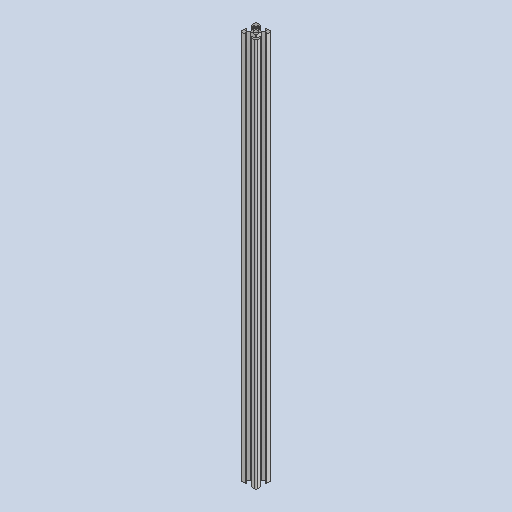
# Autodesk Inventor part: HCMUTE-CDT23-OP_NDH-2020X500
Saved by Autodesk Inventor 2023 (Build 270158000, 158)
## iProperties
Created: 2023-11-14
Part Number: HCMUTE-CDT23-OP_NDH-2020X500
Material: Generic
Document SubType Name: Modeling
Designer: havie
Density: 1 g/cm^3
Appearance: Default
Author: havie
Autodesk Inventor part; units mm, degrees
ref_plane "YZ Plane" through (0, 0, 0) normal (1, 0, 0) x (0, 1, 0)
ref_plane "XZ Plane" through (0, 0, 0) normal (0, 1, 0) x (-1, 0, 0)
ref_plane "XY Plane" through (0, 0, 0) normal (0, 0, 1) x (1, 0, 0)
sketch "Sketch1" plane through (0, 0, 0) normal (0, 0, 1) x (1, 0, 0)
  line L0 (-8.5, 10) -> (-4.1, 10)
  line L1 (10, 10) -> (10, -10)
  line L2 (10, -10) -> (-10, -10)
  line L3 (-10, 4.1) -> (-10, 8.5)
  line L4 (-10, 10) -> (10, -10) construction
  line L5 (10, 10) -> (-10, -10) construction
  line L6 (2.9101, 3.9) -> (-2.9101, 3.9)
  line L7 (-3.9, 2.9101) -> (-3.9, -2.9101)
  line L8 (3.9, -2.9101) -> (3.9, 2.9101)
  line L9 (-3.1, 9) -> (-3.1, 8.7)
  line L10 (-3.6, 8.2) -> (-5, 8.2)
  line L11 (-5.5, 7.7) -> (-5.5, 6.4899)
  line L12 (-8.2, 5) -> (-8.2, 3.6)
  line L13 (-8.7, 3.1) -> (-9, 3.1)
  line L14 (-7.7, 5.5) -> (-6.4899, 5.5)
  arc A0 (-8.5, 10) -> (-10, 8.5) centre (-8.5, 8.5) ccw
  line L15 (-3.6, 9.5) -> (-3.6, 9.5)
  line L16 (-3.6, 9.5) -> (-3.6, 9.5)
  line L17 (-9.5, 3.6) -> (-9.5, 3.6)
  line L18 (-9.5, 3.6) -> (-9.5, 3.6)
  arc A1 (-5, 8.2) -> (-5.5, 7.7) centre (-5, 7.7) ccw
  arc A2 (-7.7, 5.5) -> (-8.2, 5) centre (-7.7, 5) ccw
  arc A3 (-8.7, 3.1) -> (-8.2, 3.6) centre (-8.7, 3.6) ccw
  arc A4 (-3.6, 8.2) -> (-3.1, 8.7) centre (-3.6, 8.7) ccw
  arc A5 (-3.1, 9) -> (-3.6, 9.5) centre (-3.6, 9) ccw
  arc A6 (-3.6, 9.5) -> (-4.1, 10) centre (-4.1, 9.5) ccw
  arc A7 (-9.5, 3.6) -> (-9, 3.1) centre (-9, 3.6) ccw
  arc A8 (-10, 4.1) -> (-9.5, 3.6) centre (-9.5, 4.1) ccw
  line L19 (-6.4899, 5.5) -> (-3.9, 2.9101)
  line L20 (-5.5, 6.4899) -> (-2.9101, 3.9)
  line L21 (-14.4349, 0) -> (14.4349, 0) construction
  line L22 (0, -14.4349) -> (0, 14.4349) construction
  line L23 (8.5, 10) -> (4.1, 10)
  line L24 (10, 4.1) -> (10, 8.5)
  line L25 (3.1, 9) -> (3.1, 8.7)
  line L26 (3.6, 8.2) -> (5, 8.2)
  line L27 (5.5, 7.7) -> (5.5, 6.4899)
  line L28 (8.2, 5) -> (8.2, 3.6)
  line L29 (8.7, 3.1) -> (9, 3.1)
  line L30 (7.7, 5.5) -> (6.4899, 5.5)
  arc A9 (10, 8.5) -> (8.5, 10) centre (8.5, 8.5) ccw
  line L31 (3.6, 9.5) -> (3.6, 9.5)
  line L32 (3.6, 9.5) -> (3.6, 9.5)
  line L33 (9.5, 3.6) -> (9.5, 3.6)
  line L34 (9.5, 3.6) -> (9.5, 3.6)
  arc A10 (5.5, 7.7) -> (5, 8.2) centre (5, 7.7) ccw
  arc A11 (8.2, 5) -> (7.7, 5.5) centre (7.7, 5) ccw
  arc A12 (8.2, 3.6) -> (8.7, 3.1) centre (8.7, 3.6) ccw
  arc A13 (3.1, 8.7) -> (3.6, 8.2) centre (3.6, 8.7) ccw
  arc A14 (3.6, 9.5) -> (3.1, 9) centre (3.6, 9) ccw
  arc A15 (4.1, 10) -> (3.6, 9.5) centre (4.1, 9.5) ccw
  arc A16 (9, 3.1) -> (9.5, 3.6) centre (9, 3.6) ccw
  arc A17 (9.5, 3.6) -> (10, 4.1) centre (9.5, 4.1) ccw
  line L35 (6.4899, 5.5) -> (3.9, 2.9101)
  line L36 (5.5, 6.4899) -> (2.9101, 3.9)
  line L37 (-8.5, -10) -> (-4.1, -10)
  line L38 (-10, -4.1) -> (-10, -8.5)
  line L39 (-3.1, -9) -> (-3.1, -8.7)
  line L40 (-3.6, -8.2) -> (-5, -8.2)
  line L41 (-5.5, -7.7) -> (-5.5, -6.4899)
  line L42 (-8.2, -5) -> (-8.2, -3.6)
  line L43 (-8.7, -3.1) -> (-9, -3.1)
  line L44 (-7.7, -5.5) -> (-6.4899, -5.5)
  arc A18 (-10, -8.5) -> (-8.5, -10) centre (-8.5, -8.5) ccw
  arc A19 (-5.5, -7.7) -> (-5, -8.2) centre (-5, -7.7) ccw
  arc A20 (-8.2, -5) -> (-7.7, -5.5) centre (-7.7, -5) ccw
  arc A21 (-8.2, -3.6) -> (-8.7, -3.1) centre (-8.7, -3.6) ccw
  arc A22 (-3.1, -8.7) -> (-3.6, -8.2) centre (-3.6, -8.7) ccw
  arc A23 (-3.6, -9.5) -> (-3.1, -9) centre (-3.6, -9) ccw
  arc A24 (-4.1, -10) -> (-3.6, -9.5) centre (-4.1, -9.5) ccw
  arc A25 (-9, -3.1) -> (-9.5, -3.6) centre (-9, -3.6) ccw
  arc A26 (-9.5, -3.6) -> (-10, -4.1) centre (-9.5, -4.1) ccw
  line L45 (-6.4899, -5.5) -> (-3.9, -2.9101)
  line L46 (-5.5, -6.4899) -> (-2.9101, -3.9)
  arc A27 (10, -4.1) -> (9.5, -3.6) centre (9.5, -4.1) ccw
  line L47 (6.4899, -5.5) -> (3.9, -2.9101)
  arc A28 (7.7, -5.5) -> (8.2, -5) centre (7.7, -5) ccw
  line L48 (5.5, -7.7) -> (5.5, -6.4899)
  line L49 (10, -4.1) -> (10, -8.5)
  line L50 (3.1, -9) -> (3.1, -8.7)
  line L51 (8.5, -10) -> (4.1, -10)
  line L52 (3.6, -8.2) -> (5, -8.2)
  arc A29 (5, -8.2) -> (5.5, -7.7) centre (5, -7.7) ccw
  line L53 (7.7, -5.5) -> (6.4899, -5.5)
  arc A30 (8.7, -3.1) -> (8.2, -3.6) centre (8.7, -3.6) ccw
  arc A31 (8.5, -10) -> (10, -8.5) centre (8.5, -8.5) ccw
  line L54 (8.2, -5) -> (8.2, -3.6)
  line L55 (8.7, -3.1) -> (9, -3.1)
  arc A32 (9.5, -3.6) -> (9, -3.1) centre (9, -3.6) ccw
  arc A33 (3.6, -8.2) -> (3.1, -8.7) centre (3.6, -8.7) ccw
  arc A34 (3.1, -9) -> (3.6, -9.5) centre (3.6, -9) ccw
  arc A35 (3.6, -9.5) -> (4.1, -10) centre (4.1, -9.5) ccw
  line L56 (5.5, -6.4899) -> (2.9101, -3.9)
  line L57 (-2.9101, -3.9) -> (2.9101, -3.9)
  circle A36 centre (0, 0) radius 2.5
  point P0 (-9.5, 3.1)
  point P1 (-3.6, 9.5)
  point P2 (-3.6, 9.5)
  point P3 (-10, 3.6)
  point P4 (9.5, 3.1)
  point P5 (3.6, 9.5)
  point P6 (3.6, 9.5)
  point P7 (10, 3.6)
  point P8 (-9.5, -3.1)
  point P9 (-3.6, -9.5)
  point P10 (-3.6, -9.5)
  point P11 (-3.6, -9.5)
  point P12 (-9.5, -3.6)
  point P13 (-10, -3.6)
  point P14 (10, -3.6)
  point P15 (3.6, -9.5)
  point P16 (3.6, -9.5)
  point P17 (9.5, -3.1)
  point P18 (3.6, -9.5)
  point P19 (9.5, -3.6)
  dimension "d0" = 20
  dimension "d1" = 20
  dimension "d2" = 6.1
  dimension "d3" = 1.8
  dimension "d4" = 1.8
  dimension "d5" = 6.9
  dimension "d6" = 6.9
  dimension "d7" = 4.5
  dimension "d8" = 1.5
  dimension "d9" = 0.5
  dimension "d10" = 0.5
  dimension "d11" = 0.5
  dimension "d12" = 0.5
  dimension "d13" = 0.5
  dimension "d14" = 0.5
  dimension "d15" = 0.5
  dimension "d16" = 1.4
  dimension "d17" = 0.7
  dimension "d20" = 4.5
  dimension "d22" = 6.1
  dimension "d23" = 5
  constraints: 112 end point, 111 symmetric about line, 72 point on circle, 37 centre point, 23 point on line, 18 tangent, 8 perpendicular, 5 equal radius, 5 parallel, 4 midpoint, 3 vertical, 2 horizontal, 1 coincident, 1 horizontal alignment, 27 other
  measures "d0" distance of L1.end L2.end
  measures "d1" distance of L1.start L1.end
  measures "d2" distance from line of L6.end L0
  measures "d3" distance between parallel lines of L0 L10
  measures "d4" distance between parallel lines of L3 L12
  measures "d5" distance between parallel lines of L9 L3
  measures "d6" distance between parallel lines of L13 L0
  measures "d7" distance between parallel lines of L3 L11
  measures "d8" radius of A0
  measures "d9" distance from line of L9 point (-3.6, 9.5)
  measures "d10" distance from line of L0 point (-3.6, 9.5)
  measures "d11" distance of point (-9.5, 3.1) L17.end
  measures "d12" distance of L17.end point (-10, 3.6)
  measures "d13" radius of A1
  measures "d14" radius of A5
  measures "d15" radius of A7
  measures "d16" distance between parallel lines of L20 L19
  measures "d17" distance between parallel lines of L4 L20
  measures "d20" distance between parallel lines of L0 L14
  measures "d22" distance between parallel lines of L7 L3
  measures "d23" diameter of A36
extrude "Extrusion1" add sketch "Sketch1" along normal mid plane 500 contours L0 A6 A5 L9 A4 L10 A1 L11 L20 L6 L36 L27 A10 L26 A13 L25 A14 A15 L23 A9 L1 A17 A16 L29 A12 L28 A11 L30 L35 L8 L47 L53 A28 L54 A30 L55 A32 A27 A31 L2 A35 A34 L50 A33 L52 A29 L48 L56 L57 L46 L41 A19 L40 A22 L39 A23 A24 A18 L38 A26 A25 L43 A21 L42 A20 L44 L45 L7 L19 L14 A2 L12 A3 L13 A7 A8 L3 A0
equation "\"d4\" = d3"
equation "\"d6\" = d5"
equation "\"d10\" = d9"
equation "\"d12\" = d11"
body "Solid1"
